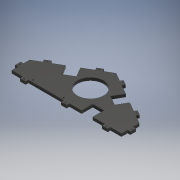
# Autodesk Inventor part: BA07
Saved by Autodesk Inventor 2017 (Build 210142000, 142)
## iProperties
Created: 2019-05-24
Part Number: BA07
Material: Wood (Cherry)
Document SubType Name: Modeling
Designer: Dell
Density: 0.63 g/cm^3
Appearance: Smooth - Black
Mass: 485.361 g
Surface Area: 1502.67 cm^2
Volume: 770.414 cm^3
Author: Dell
Autodesk Inventor part; units mm, degrees
ref_plane "YZ Plane" through (0, 0, 0) normal (1, 0, 0) x (0, 1, 0)
ref_plane "XZ Plane" through (0, 0, 0) normal (0, 1, 0) x (-1, 0, 0)
ref_plane "XY Plane" through (0, 0, 0) normal (0, 0, 1) x (1, 0, 0)
sketch "Sketch1" plane through (0, 0, 0) normal (0, 0, 1) x (1, 0, 0)
  line L0 (0, 0) -> (0, 101.6)
  line L1 (0, 0) -> (525.78, 0)
  line L2 (525.78, 0) -> (525.78, 101.6)
  line L3 (525.78, 101.6) -> (262.89, 253.3796)
  line L4 (262.89, 253.3796) -> (0, 101.6)
  line L5 (12.7, 94.2677) -> (12.7, 12.7)
  line L6 (12.7, 12.7) -> (513.08, 12.7)
  line L7 (513.08, 12.7) -> (513.08, 94.2677)
  line L8 (513.08, 94.2677) -> (262.89, 238.7149)
  line L9 (262.89, 238.7149) -> (12.7, 94.2677)
  point P0 (262.89, 0)
  dimension "d0" = 101.6
  dimension "d1" = 525.78
  dimension "d2" = 120
  dimension "d3" = 12.7
  constraints: 20 end point, 2 perpendicular, 1 horizontal, 1 horizontal alignment, 1 midpoint, 1 vertical, 1 vertical alignment, 4 other
  measures "d0" distance of L0.start L0.end
  measures "d1" distance of L0.start L1.end
  measures "d2" angle of L0 L4
  measures "d3" distance between parallel lines of L4 L9
extrude "Extrusion1" add sketch "Sketch1" along normal blind 12.7 contours L9 L8 L7 L6 L5
sketch "Sketch2" plane through (0, 0, 12.7) normal (0, 0, 1) x (1, 0, 0)
  line L0 (12.7, 94.2677) -> (12.7, 12.7) projected
  line L1 (12.7, 66.1838) -> (0, 66.1838)
  line L2 (0, 66.1838) -> (0, 40.7838)
  line L3 (0, 40.7838) -> (12.7, 40.7838)
  line L4 (12.7, 40.7838) -> (12.7, 66.1838)
  line L5 (513.08, 66.1838) -> (525.78, 66.1838)
  line L6 (525.78, 66.1838) -> (525.78, 40.7838)
  line L7 (525.78, 40.7838) -> (513.08, 40.7838)
  line L8 (513.08, 40.7838) -> (513.08, 66.1838)
  line L9 (513.08, 12.7) -> (513.08, 94.2677) projected
  line L10 (12.7, 12.7) -> (513.08, 12.7) projected
  line L11 (62.69, 12.7) -> (88.09, 12.7)
  line L12 (88.09, 12.7) -> (88.09, 0)
  line L13 (88.09, 0) -> (62.69, 0)
  line L14 (62.69, 0) -> (62.69, 12.7)
  line L15 (250.19, 12.7) -> (275.59, 12.7)
  line L16 (275.59, 12.7) -> (275.59, 0)
  line L17 (275.59, 0) -> (250.19, 0)
  line L18 (250.19, 0) -> (250.19, 12.7)
  line L19 (437.69, 12.7) -> (463.09, 12.7)
  line L20 (463.09, 12.7) -> (463.09, 0)
  line L21 (463.09, 0) -> (437.69, 0)
  line L22 (437.69, 0) -> (437.69, 12.7)
  line L23 (75.39, 0) -> (450.39, 0) construction
  line L24 (51.0193, 116.3913) -> (44.6693, 127.3898)
  line L25 (44.6693, 127.3898) -> (66.6663, 140.0898)
  line L26 (66.6663, 140.0898) -> (73.0163, 129.0913)
  line L27 (73.0163, 129.0913) -> (51.0193, 116.3913)
  line L28 (202.5737, 203.8913) -> (196.2237, 214.8898)
  line L29 (196.2237, 214.8898) -> (218.2207, 227.5898)
  line L30 (218.2207, 227.5898) -> (224.5707, 216.5913)
  line L31 (224.5707, 216.5913) -> (202.5737, 203.8913)
  line L32 (262.89, 238.7149) -> (12.7, 94.2677) projected
  line L33 (55.6678, 133.7398) -> (207.2222, 221.2398) construction
  line L34 (131.445, 177.4898) -> (137.795, 166.4913)
  line L35 (513.08, 94.2677) -> (262.89, 238.7149) projected
  line L36 (262.89, 238.7149) -> (262.89, 274.3369)
  line L37 (474.7607, 116.3913) -> (481.1107, 127.3898)
  line L38 (481.1107, 127.3898) -> (459.1137, 140.0898)
  line L39 (459.1137, 140.0898) -> (452.7637, 129.0913)
  line L40 (452.7637, 129.0913) -> (474.7607, 116.3913)
  line L41 (323.2063, 203.8913) -> (329.5563, 214.8898)
  line L42 (329.5563, 214.8898) -> (307.5593, 227.5898)
  line L43 (307.5593, 227.5898) -> (301.2093, 216.5913)
  line L44 (301.2093, 216.5913) -> (323.2063, 203.8913)
  line L45 (470.1122, 133.7398) -> (318.5578, 221.2398) construction
  line L46 (394.335, 177.4898) -> (387.985, 166.4913)
  circle A0 centre (519.43, 53.4838) radius 2.25
  circle A1 centre (466.9372, 128.2405) radius 2.25
  circle A2 centre (450.39, 6.35) radius 2.25
  circle A3 centre (262.89, 6.35) radius 2.25
  circle A4 centre (75.39, 6.35) radius 2.25
  circle A5 centre (6.35, 53.4838) radius 2.25
  circle A6 centre (58.8428, 128.2405) radius 2.25
  circle A7 centre (210.3972, 215.7405) radius 2.25
  circle A8 centre (315.3828, 215.7405) radius 2.25
  line L47 (58.8428, 128.2405) -> (55.6678, 133.7398) construction
  line L48 (58.8428, 128.2405) -> (69.8413, 134.5905) construction
  line L49 (199.3987, 209.3905) -> (210.3972, 215.7405) construction
  line L50 (210.3972, 215.7405) -> (207.2222, 221.2398) construction
  line L51 (326.3813, 209.3905) -> (315.3828, 215.7405) construction
  line L52 (315.3828, 215.7405) -> (318.5578, 221.2398) construction
  line L53 (455.9387, 134.5905) -> (466.9372, 128.2405) construction
  line L54 (466.9372, 128.2405) -> (470.1122, 133.7398) construction
  point P0 (0, 0)
  point P1 (12.7, 53.4838)
  point P2 (513.08, 53.4838)
  point P3 (262.89, 12.7)
  point P4 (262.89, 0)
  point P5 (262.89, 12.7)
  point P6 (88.09, 6.35)
  point P7 (250.19, 6.35)
  point P8 (437.69, 6.35)
  point P9 (12.7, 53.4838)
  point P10 (6.35, 66.1838)
  point P11 (75.39, 12.7)
  point P12 (262.89, 12.7)
  point P13 (450.39, 12.7)
  point P14 (519.43, 66.1838)
  dimension "d6" = 12.7
  dimension "d7" = 25.4
  dimension "d8" = 12.7
  dimension "d9" = 25.4
  dimension "d10" = 25.4
  dimension "d11" = 12.7
  dimension "d12" = 25.4
  dimension "d13" = 12.7
  dimension "d14" = 25.4
  dimension "d15" = 12.7
  dimension "d16" = 375
  dimension "d17" = 25.4
  dimension "d18" = 12.7
  dimension "d19" = 12.7
  dimension "d20" = 25.4
  dimension "d21" = 175
  dimension "d28" = 4.5
  dimension "d29" = 4.5
  dimension "d30" = 4.5
  dimension "d31" = 4.5
  dimension "d32" = 4.5
  dimension "d33" = 4.5
  dimension "d34" = 4.5
  dimension "d35" = 4.5
  dimension "d36" = 4.5
  constraints: 100 end point, 24 midpoint, 16 perpendicular, 14 parallel, 12 symmetric about line, 9 centre point, 6 point on line, 6 vertical alignment, 5 horizontal, 5 horizontal alignment, 1 vertical, 8 other
  measures "d6" distance of L3.end L2.end
  measures "d7" distance of L2.end L1.end
  measures "d8" distance of L6.end L7.end
  measures "d9" distance of L5.end L6.end
  measures "d10" distance of L12.end L13.end
  measures "d11" distance of L11.end L12.end
  measures "d12" distance of L16.end L17.end
  measures "d13" distance of L15.end L16.end
  measures "d14" distance of L20.end L21.end
  measures "d15" distance of L19.end L20.end
  measures "d16" distance of L23.start L23.end
  measures "d17" distance of L28.end L29.end
  measures "d18" distance of L29.end L30.end
  measures "d19" distance of L24.start L24.end
  measures "d20" distance of L24.end L25.end
  measures "d21" distance of L33.start L33.end
  measures "d28" diameter of A0
  measures "d29" diameter of A1
  measures "d30" diameter of A2
  measures "d31" diameter of A3
  measures "d32" diameter of A4
  measures "d33" diameter of A5
  measures "d34" diameter of A6
  measures "d35" diameter of A7
  measures "d36" diameter of A8
extrude "Extrusion2" add sketch "Sketch2" against normal blind 12.7
sketch "Sketch3" plane through (0, 0, 12.7) normal (0, 0, 1) x (1, 0, 0)
  circle A0 centre (262.89, 121.3796) radius 60
  line L0 (250.19, 0) -> (275.59, 0) projected
  point P0 (0, 0)
  point P1 (262.89, 0)
  dimension "d24" = 120
  dimension "d25" = 121.3796
  constraints: 1 centre point, 1 midpoint, 1 vertical alignment
  measures "d24" diameter of A0
  measures "d25" distance from line of L0 A0.centre
extrude "Extrusion3" cut sketch "Sketch3" against normal through all
sketch "Sketch5" plane through (0, 0, 12.7) normal (0, 0, 1) x (1, 0, 0)
  line L0 (275.59, 12.7) -> (437.69, 12.7) projected
  line L1 (331.24, 12.7) -> (382.04, 12.7)
  line L2 (382.04, 12.7) -> (382.04, 63.5)
  line L3 (382.04, 63.5) -> (331.24, 63.5)
  line L4 (331.24, 63.5) -> (331.24, 12.7)
  point P0 (0, 0)
  point P1 (356.64, 12.7)
  dimension "d37" = 50.8
  dimension "d38" = 50.8
  constraints: 8 end point, 2 midpoint, 2 parallel, 1 horizontal, 1 perpendicular, 1 point on line
  measures "d37" distance of L3.end L2.end
  measures "d38" distance of L2.end L1.end
extrude "Extrusion4" cut sketch "Sketch5" against normal through all
sketch "Sketch6" plane through (0, 0, 12.7) normal (0, 0, 1) x (1, 0, 0)
  line L0 (159.792, 179.1913) -> (185.192, 135.1972)
  line L1 (185.192, 135.1972) -> (141.198, 109.7972)
  line L2 (141.198, 109.7972) -> (115.798, 153.7913)
  line L3 (115.798, 153.7913) -> (159.792, 179.1913)
  line L4 (452.7637, 129.0913) -> (323.2063, 203.8913) projected
  line L5 (409.982, 153.7913) -> (384.582, 109.7972)
  line L6 (384.582, 109.7972) -> (340.588, 135.1972)
  line L7 (340.588, 135.1972) -> (365.988, 179.1913)
  line L8 (365.988, 179.1913) -> (409.982, 153.7913)
  line L9 (202.5737, 203.8913) -> (73.0163, 129.0913) projected
  point P0 (0, 0)
  point P1 (137.795, 166.4913)
  point P2 (387.985, 166.4913)
  dimension "d41" = 50.8
  dimension "d42" = 50.8
  dimension "d43" = 50.8
  dimension "d44" = 50.8
  constraints: 16 end point, 4 midpoint, 4 parallel, 4 point on line, 2 perpendicular
  measures "d41" distance of L5.end L6.end
  measures "d42" distance of L5.start L5.end
  measures "d43" distance of L0.end L1.end
  measures "d44" distance of L0.start L0.end
extrude "Extrusion5" cut sketch "Sketch6" against normal through all
sketch "Sketch7" plane through (0, 0, 12.7) normal (0, 0, 1) x (1, 0, 0)
  line L0 (88.09, 12.7) -> (110.19, 12.7) construction
  line L1 (110.19, 12.7) -> (110.19, 32.7) construction
  line L2 (110.19, 32.7) -> (88.09, 32.7) construction
  line L3 (88.09, 32.7) -> (88.09, 12.7) construction
  line L4 (250.19, 12.7) -> (228.09, 12.7) construction
  line L5 (228.09, 12.7) -> (228.09, 32.7) construction
  line L6 (228.09, 32.7) -> (250.19, 32.7) construction
  line L7 (250.19, 32.7) -> (250.19, 12.7) construction
  circle A0 centre (99.14, 22.7) radius 3
  circle A1 centre (239.14, 22.7) radius 3
  point P0 (0, 0)
  point P1 (99.14, 32.7)
  point P2 (239.14, 32.7)
  point P3 (88.09, 22.7)
  point P4 (250.19, 22.7)
  dimension "d48" = 20
  dimension "d50" = 20
  dimension "d51" = 6
  dimension "d52" = 6
  dimension "d55" = 11.05
  dimension "d56" = 11.05
  constraints: 16 end point, 4 midpoint, 4 parallel, 3 coincident, 2 centre point, 2 horizontal, 2 horizontal alignment, 2 perpendicular, 2 vertical alignment, 1 point on line
  measures "d48" distance of L1.end L0.end
  measures "d50" distance of L4.end L5.end
  measures "d51" diameter of A0
  measures "d52" diameter of A1
  measures "d55" horizontal distance of point (88.09, 12.7) A0.centre
  measures "d56" horizontal distance of A1.centre point (250.19, 12.7)
extrude "Extrusion6" cut sketch "Sketch7" against normal through all
equation "\"d6\" = d11"
equation "\"d8\" = d11"
equation "\"d13\" = d11"
equation "\"d15\" = d13"
equation "\"d18\" = d11"
equation "\"d19\" = d11"
body "Solid1"
